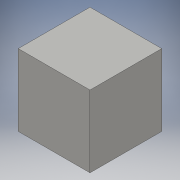
# Autodesk Inventor part: Block
Saved by Autodesk Inventor 2016 (Build 200138000, 138)
## iProperties
Created: 2015-09-10
Part Number: Block
Material: Generic
Document SubType Name: Modeling
Designer: Kiran
Density: 1 g/cm^3
Appearance: Default
Mass: 125 g
Surface Area: 150 cm^2
Volume: 125 cm^3
Author: Kiran
Autodesk Inventor part; units mm, degrees
ref_plane "YZ Plane" through (0, 0, 0) normal (1, 0, 0) x (0, 1, 0)
ref_plane "XZ Plane" through (0, 0, 0) normal (0, 1, 0) x (-1, 0, 0)
ref_plane "XY Plane" through (0, 0, 0) normal (0, 0, 1) x (1, 0, 0)
sketch "Sketch2" plane through (0, 0, 0) normal (0, 1, 0) x (-1, 0, 0)
  line L0 (0, 0) -> (-50, 0)
  line L1 (-50, 0) -> (-50, 50)
  line L2 (-50, 50) -> (0, 50)
  line L3 (0, 50) -> (0, 0)
  dimension "d4" = 50
  dimension "d5" = 50
  constraints: 8 end point, 2 parallel, 1 horizontal, 1 perpendicular
  measures "d4" distance of L0.start L0.end
  measures "d5" distance of L0.end L1.end
extrude "Extrusion2" add sketch "Sketch2" along normal blind 50
body "Solid2"
